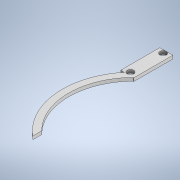
# Autodesk Inventor part: grabber
Saved by Autodesk Inventor 2021 (Build 250183000, 183)
## iProperties
Created: 2021-01-01
Part Number: grabber
Material: Generic
Document SubType Name: Modeling
Designer: gabe3
Density: 1 g/cm^3
Appearance: Default
Author: gabe3
Autodesk Inventor part; units mm, degrees
ref_plane "YZ Plane" through (0, 0, 0) normal (1, 0, 0) x (0, 1, 0)
ref_plane "XZ Plane" through (0, 0, 0) normal (0, 1, 0) x (-1, 0, 0)
ref_plane "XY Plane" through (0, 0, 0) normal (0, 0, 1) x (1, 0, 0)
sketch "Sketch1" plane through (0, 0, 0) normal (0, 1, 0) x (-1, 0, 0)
  arc A0 (44.7326, -45.0693) -> (44.7326, 45.0693) centre (0, 0) ccw
  line L0 (44.6636, -44.4546) -> (57.3636, -44.4546)
  line L1 (57.3636, -44.4546) -> (57.3636, -82.5546)
  line L2 (57.3636, -82.5546) -> (44.6636, -82.5546)
  line L3 (44.6636, -82.5546) -> (44.6636, -44.4546)
  line L4 (44.7326, -53.6471) -> (44.7326, 53.6471)
  arc A1 (44.7326, -53.6471) -> (44.7326, 53.6471) centre (0, 0) ccw
  point P0 (53.8778, -44.4546)
  point P1 (45.3436, -44.4546)
  dimension "d0" = 63.5
  dimension "d2" = 12.7
  dimension "d3" = 38.1
  constraints: 10 end point, 4 point on circle, 2 centre point, 2 parallel, 2 point on line, 1 coincident, 1 horizontal, 1 perpendicular
  measures "d0" radius of A0
  measures "d2" distance of L1.end L2.end
  measures "d3" distance of L0.end L1.end
extrude "Extrusion1" add sketch "Sketch1" along normal blind 3.175 contours L4 L0 A0 | A0 L0 A1 L4 | L4 A1 L0 L1 L2 L3 | A0 L4 A1 L0 picked at (44.8008, -44.7964)
sketch "Sketch2" plane through (0, 3.175, 0) normal (0, 1, 0) x (1, 0, 0)
  line L0 (-57.3636, 82.5546) -> (-57.3636, 44.4546) projected
  line L1 (-44.6636, 82.5546) -> (-57.3636, 82.5546) projected
  line L2 (-45.3436, 44.4546) -> (-44.6636, 44.4546) projected
  line L3 (-44.6636, 44.4546) -> (-44.6636, 82.5546) projected
  line L4 (-57.3636, 44.4546) -> (-53.8778, 44.4546) projected
  arc A0 (-53.8778, 44.4546) -> (-44.7326, -53.6471) centre (0, 0) ccw projected
  line L5 (-44.7326, -53.6471) -> (-44.7326, -45.0693) projected
  arc A1 (-45.3436, 44.4546) -> (-44.7326, -45.0693) centre (0, 0) ccw projected
  point P0 (-51.0136, 47.6296)
  point P1 (-51.0136, 79.3796)
  dimension "d6" = 12.7
  dimension "d7" = 6.35
  dimension "d8" = 6.35
  dimension "d9" = 31.75
  dimension "d10" = 38.1
  dimension "d11" = 3.175
  measures "d6" distance of L1.start L0.start
  measures "d7" distance from line of L0 point (-51.014, 79.38)
  measures "d8" distance from line of L0 point (-51.014, 47.63)
  measures "d9" distance of point (-51.014, 79.38) point (-51.014, 47.63)
  measures "d10" distance of L2.end L1.start
  measures "d11" distance from line of L1 point (-51.014, 79.38)
hole "Hole1" at (-51.0136, 3.175, -47.6296) at (-51.0136, 3.175, -79.3796) direction (0, -1, 0) diameter 6.35 depth 19.05 tip angle 118
equation "\"d7\" = 0.5 * d6"
equation "\"d8\" = d7"
equation "\"d11\" = -0.5 * d9 + 0.5 * d10"
body "Solid1"
